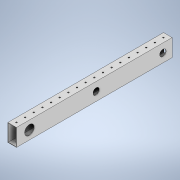
# Autodesk Inventor part: VerseFrame 18in Uptake
Saved by Autodesk Inventor 2021 (Build 250183000, 183)
## iProperties
Created: 2021-03-02
Part Number: VerseFrame 18in Uptake
Material: Generic
Document SubType Name: Modeling
Designer: Merkileg
Density: 1 g/cm^3
Appearance: Default
Author: Merkileg
Autodesk Inventor part; units mm, degrees
ref_plane "YZ Plane" through (0, 0, 0) normal (1, 0, 0) x (0, 1, 0)
ref_plane "XZ Plane" through (0, 0, 0) normal (0, 1, 0) x (-1, 0, 0)
ref_plane "XY Plane" through (0, 0, 0) normal (0, 0, 1) x (1, 0, 0)
sketch "Sketch1" plane through (0, 0, 0) normal (0, 0, 1) x (1, 0, 0)
  line L0 (0, 0) -> (25.4, 0)
  line L1 (25.4, 0) -> (25.4, 50.8)
  line L2 (25.4, 50.8) -> (0, 50.8)
  line L3 (0, 50.8) -> (0, 0)
  line L4 (1.27, 1.27) -> (24.13, 1.27)
  line L5 (24.13, 1.27) -> (24.13, 49.53)
  line L6 (24.13, 49.53) -> (1.27, 49.53)
  line L7 (1.27, 49.53) -> (1.27, 1.27)
  dimension "d0" = 25.4
  dimension "d1" = 50.8
  dimension "d4" = 1.27
  dimension "d5" = 1.27
  constraints: 16 end point, 4 parallel, 2 horizontal, 2 perpendicular
  measures "d0" distance of L2.end L1.end
  measures "d1" distance of L1.end L0.end
  measures "d4" distance between parallel lines of L1 L5
  measures "d5" distance between parallel lines of L0 L4
extrude "Extrusion1" add sketch "Sketch1" along normal blind 457.2
sketch "Sketch2" plane through (0, 50.8, 0) normal (0, 1, 0) x (1, 0, 0)
  line L0 (1.27, -457.2) -> (24.13, -457.2) projected
  circle A0 centre (12.7, -12.7) radius 2.0701
  line L1 (0, 0) -> (0, -457.2) projected
  line L2 (25.4, 0) -> (0, 0) projected
  dimension "d9" = 4.1402
  dimension "d10" = 12.7
  dimension "d11" = 12.7
  constraints: 1 centre point
  measures "d9" diameter of A0
  measures "d10" distance from line of L1 A0.centre
  measures "d11" distance from line of L2 A0.centre
extrude "Extrusion2" cut sketch "Sketch2" against normal blind 457.2
pattern_linear "Rectangular Pattern1" count 18 spacing 25.4 along (0, 0, 1) of "Extrusion2"
sketch "Sketch3" plane through (25.4, 0, 0) normal (1, 0, 0) x (0, 0, -1)
  line L0 (-457.2, 0) -> (-457.2, 50.8) projected
  line L1 (-457.2, 25.4) -> (0, 25.4) construction
  circle A0 centre (-419.1, 25.4) radius 14.2875
  circle A1 centre (-223.1482, 25.4) radius 9.525
  circle A2 centre (-27.1964, 25.4) radius 9.525
  point P0 (0, 0)
  dimension "d17" = 19.05
  dimension "d18" = 38.1
  dimension "d19" = 28.575
  dimension "d20" = 195.9518
  dimension "d21" = 195.9518
  constraints: 3 centre point, 3 point on line, 2 end point, 1 equal radius, 1 horizontal, 1 midpoint
  measures "d17" diameter of A1
  measures "d18" distance from line of L0 A0.centre
  measures "d19" diameter of A0
  measures "d20" distance of A1.centre A0.centre
  measures "d21" distance of A2.centre A1.centre
extrude "Extrusion3" cut sketch "Sketch3" against normal through all
equation "\"d0\" = u1"
equation "\"d1\" = u2"
equation "\"d4\" = u3"
equation "\"d5\" = u3"
equation "\"d6\" = u4"
equation "\"d9\" = u5"
equation "\"d10\" = u6"
equation "\"d11\" = u7"
equation "\"d12\" = u4"
equation "\"d20\" = u10"
equation "\"d21\" = u10"
equation "\"d16\" = u9"
equation "\"u1\" = 25.4"
equation "\"u2\" = 50.8"
equation "\"u3\" = 1.27"
equation "\"u4\" = 457.2"
equation "\"u5\" = 4.1402"
equation "\"u6\" = 12.7"
equation "\"u7\" = 12.7"
equation "\"u9\" = 25.4"
equation "\"u10\" = 195.95178"
body "Solid1"
